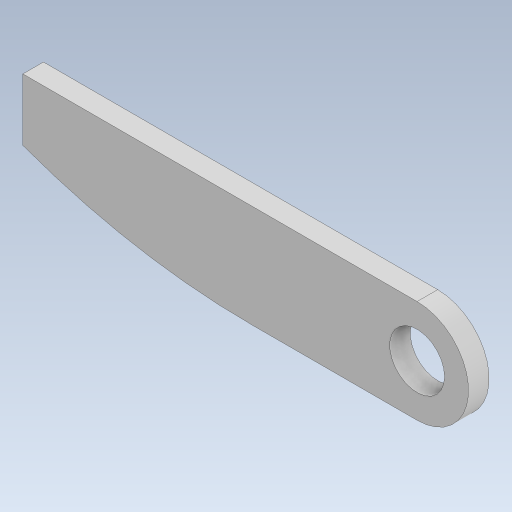
# Autodesk Inventor part: 零件6
Saved by Autodesk Inventor 2023 (Build 270158000, 158)
## iProperties
Created: 2023-05-12
Part Number: 零件6
Material: 一般
Document SubType Name: Modeling
Designer: Johnny Jou
Density: 1 g/cm^3
Appearance: 預設
Author: Johnny Jou
Autodesk Inventor part; units mm, degrees
ref_plane "YZ Plane" through (0, 0, 0) normal (1, 0, 0) x (0, 1, 0)
ref_plane "XZ Plane" through (0, 0, 0) normal (0, 1, 0) x (-1, 0, 0)
ref_plane "XY Plane" through (0, 0, 0) normal (0, 0, 1) x (1, 0, 0)
sketch "草圖1" plane through (0, 0, 0) normal (0, 0, 1) x (1, 0, 0)
  line L0 (0, 0) -> (50, 0)
  line L1 (50, 0) -> (50, 15)
  line L2 (50, 15) -> (0, 15)
  line L3 (0, 15) -> (0, 0)
  circle A0 centre (57.5, 7.5) radius 7.5
  line L4 (50, 15) -> (57.5, 15)
  line L5 (50, 0) -> (57.5, 0)
  circle A1 centre (57.5, 7.5) radius 4
  arc A2 (-63.5, 97) -> (33.5, 0) centre (33.5, 97) ccw
  line L6 (33.5, 0) -> (53.5, 0)
  line L7 (53.5, 7.5) -> (53.5, 0)
  point P0 (0, 5.9684)
  point P1 (33.5, 0)
  dimension "d3" = 8
  dimension "d0" = 50
  dimension "d1" = 15
  dimension "d2" = 15
  dimension "d6" = 20
  dimension "d7" = 97
  dimension "d8" = 137.1787
  constraints: 16 end point, 5 tangent, 4 point on circle, 2 centre point, 2 parallel, 2 perpendicular, 1 coincident, 1 collinear, 1 horizontal, 1 horizontal alignment, 1 vertical, 2 other
  measures "d0" distance of L1.end L2.end
  measures "d1" distance of L0.end L1.end
  measures "d2" diameter of A0
  measures "d6" distance of L6.start L6.end
  measures "d7" radius of A2
  measures "d8" distance of L6.start A2.start
extrude "擠出1" add sketch "草圖1" along normal blind 3 contours A2 L3 L2 L1 L0 | L1 A0 L7 L5 | L1 L4 A0 | A0 | L7 A0 L5
